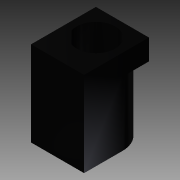
# Autodesk Inventor part: pj-002b
Saved by Autodesk Inventor 2016 (Build 200138000, 138)
## iProperties
Created: 2017-03-05
Part Number: pj-002b
Material: Generic
Document SubType Name: Modeling
Designer: Tyler
Density: 1 g/cm^3
Appearance: Smooth - Black
Author: Tyler
Autodesk Inventor part; units mm, degrees
ref_plane "YZ Plane" through (0, 0, 0) normal (1, 0, 0) x (0, 1, 0)
ref_plane "XZ Plane" through (0, 0, 0) normal (0, 1, 0) x (-1, 0, 0)
ref_plane "XY Plane" through (0, 0, 0) normal (0, 0, 1) x (1, 0, 0)
sketch "Sketch1" plane through (0, 0, 0) normal (0, 0, 1) x (1, 0, 0)
  line L0 (-4.5, 0) -> (4.5, 0)
  line L1 (4.5, 0) -> (4.5, 11)
  line L2 (4.5, 11) -> (-4.5, 11)
  line L3 (-4.5, 11) -> (-4.5, 0)
  line L4 (-4.5, 0) -> (4.5, 11) construction
  line L5 (4.5, 0) -> (-4.5, 11) construction
  point P0 (0, 0)
  point P1 (0, 5.5)
  dimension "d0" = 9
  dimension "d1" = 11
  dimension "d2" = 0
  dimension "d3" = 0
  constraints: 12 end point, 2 midpoint, 2 parallel, 1 horizontal, 1 perpendicular
  measures "d0" distance of L2.end L1.end
  measures "d1" distance of L0.end L1.end
  measures "d2" distance from line of point (0, 0) L0
  measures "d3" horizontal distance of point (0, 5.5) point (0, 0)
extrude "Extrusion1" add sketch "Sketch1" against normal blind 3.5
sketch "Sketch2" plane through (0, 0, -3.5) normal (0, 0, -1) x (-1, 0, 0)
  line L0 (-4.5, 0) -> (4.5, 0) projected
  line L1 (4.5, 0) -> (4.5, 11) projected
  line L2 (4.5, 11) -> (-4.5, 11) projected
  line L3 (-4.5, 11) -> (-4.5, 0) projected
  arc A0 (4.5, 6.5) -> (-4.5, 6.5) centre (0, 6.5) ccw
  point P0 (0, 0)
  constraints: 2 point on circle, 2 point on line, 2 tangent, 1 centre point
extrude "Extrusion2" add sketch "Sketch2" along normal blind 10.9 contours L3 A0 L1 L0
sketch "Sketch3" plane through (0, 0, 0) normal (0, 0, 1) x (1, 0, 0)
  circle A0 centre (0, 6.5) radius 3.25
  point P0 (0, 0)
  dimension "d8" = 6.5
  dimension "d9" = 6.5
  constraints: 1 centre point
  measures "d8" diameter of A0
  measures "d9" distance of point (0, 0) A0.centre
extrude "Extrusion3" cut sketch "Sketch3" against normal blind 10.9
body "Solid1"
